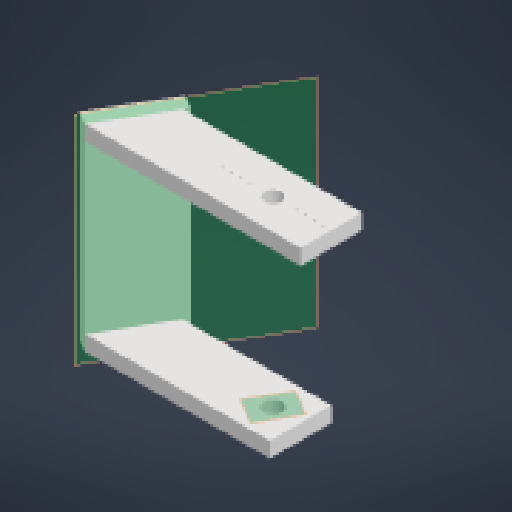
# Autodesk Inventor part: manipulator_arm
Saved by Autodesk Inventor 2024 (Build 280153000, 153)
## iProperties
Created: 2023-05-17
Part Number: manipulator_arm
Material: Типовые
Document SubType Name: Modeling
Designer: user
Density: 1 g/cm^3
Appearance: По умолчанию
Author: user
Autodesk Inventor part; units mm, degrees
ref_plane "YZ Plane" through (0, 0, 0) normal (1, 0, 0) x (0, 1, 0)
ref_plane "XZ Plane" through (0, 0, 0) normal (0, 1, 0) x (-1, 0, 0)
ref_plane "XY Plane" through (0, 0, 0) normal (0, 0, 1) x (1, 0, 0)
sketch "Эскиз1" plane through (0, 0, 0) normal (0, 0, 1) x (1, 0, 0)
  line L0 (-81, 10) -> (19, 10)
  line L1 (19, 10) -> (19, -10)
  line L2 (19, -10) -> (-81, -10)
  line L3 (-81, -10) -> (-81, 10)
  line L4 (19, 0) -> (0, 0) construction
  arc A0 (16.8881, -2.4697) -> (16.8881, 2.4697) centre (16.5, 0) ccw construction
  circle A1 centre (16.5, 0) radius 0.65 construction
  circle A2 centre (13.5, 0) radius 0.65 construction
  circle A3 centre (10.5, 0) radius 0.65 construction
  circle A4 centre (7.5, 0) radius 0.65 construction
  circle A5 centre (-7.5, 0) radius 0.65 construction
  circle A6 centre (-10.5, 0) radius 0.65 construction
  circle A7 centre (-13.5, 0) radius 0.65 construction
  circle A8 centre (-16.5, 0) radius 0.65 construction
  circle A9 centre (-16.5, 0) radius 0.4
  circle A10 centre (-13.5, 0) radius 0.4
  circle A11 centre (-10.5, 0) radius 0.4
  circle A12 centre (-7.5, 0) radius 0.4
  circle A13 centre (7.5, 0) radius 0.4
  circle A14 centre (10.5, 0) radius 0.4
  circle A15 centre (13.5, 0) radius 0.4
  circle A16 centre (16.5, 0) radius 0.4
  circle A17 centre (0, 0) radius 2.75 projected
  dimension "d0" = 20
  dimension "d3" = 100
  dimension "d28" = 0.8
  constraints: 10 end point, 8 centre point, 8 coincident, 7 equal radius, 3 perpendicular, 1 horizontal, 1 midpoint, 1 parallel, 1 tangent
  measures "d0" distance of L0.end L1.end
  measures "d3" distance of L1.end L2.end
  measures "d28" diameter of A9
extrude "Выдавливание1" add sketch "Эскиз1" along normal blind 5
ref_plane "РабПлоскость1" through (0, 0, -54.2) normal (0, 0, -1) x (-0.5, -0.8660254, 0)
sketch "Эскиз2" plane through (0, 0, -54.2) normal (0, 0, -1) x (-0.5, -0.8660254, 0)
  line L0 (31.8397, 75.1481) -> (49.1603, 65.1481) projected
  line L1 (49.1603, 65.1481) -> (4.1603, -12.7942)
  line L2 (49.1603, 65.1481) -> (-0.8397, -21.4545) projected
  line L3 (4.1603, -12.7942) -> (-13.1603, -2.7942)
  line L4 (-18.1603, -11.4545) -> (31.8397, 75.1481) projected
  line L5 (-13.1603, -2.7942) -> (31.8397, 75.1481)
  circle A0 centre (0, 0) radius 3 projected
  point P0 (0, 0)
  dimension "d4" = 90
  constraints: 6 end point, 2 point on line, 1 collinear, 1 perpendicular
  measures "d4" distance of L0.end L1.end
extrude "Выдавливание2" add sketch "Эскиз2" along normal blind 5
ref_plane "РабПлоскость3" through (-81, -10, 5) normal (-0.8660254, 0.5, 0) x (0.5, 0.8660254, 0)
ref_plane "РабПлоскость2" through (-22.6159, -10.6718, -31.45) normal (-0.8660254, 0.5, 0) x (0.5, 0.8660254, 0)
sketch "Эскиз3" plane through (-81, -10, 5) normal (-0.8660254, 0.5, 0) x (0.5, 0.8660254, 0)
  line L0 (0, 59.2) -> (17.3205, 59.2) projected
  line L1 (0, 5) -> (50, 5) projected
  line L2 (0, 59.2) -> (25, 59.2)
  line L3 (25, 59.2) -> (25, 5)
  line L4 (25, 5) -> (0, 5)
  line L5 (0, 5) -> (0, 59.2)
  point P0 (49.1603, 5)
  point P1 (0, 5)
  point P2 (17.3205, 59.2)
  dimension "d7" = 25
  constraints: 8 end point, 2 parallel, 1 horizontal, 1 midpoint, 1 perpendicular
  measures "d7" distance of L1.start L3.end
extrude "Выдавливание3" add sketch "Эскиз3" along normal blind 5
move faces "Перенос1" translate (0, 0, 5) faces at (-82.4434, -5.8333, 0)
move faces "Перенос2" translate (0, 0, -5) faces at (-82.4434, -5.8333, -54.2)
move faces "Перенос3" translate (0, 0, -6.5) faces at (-79.0755, 6.6667, -54.2)
move faces "Перенос4" translate (0, 0, 7.5) faces at (-79.0755, 6.6667, 0)
move faces "Перенос5" translate (0, 0, 5) faces at (-72.5032, 11.3835, 0)
move faces "Перенос6" translate (0, 0, -5) faces at (-72.5032, 11.3835, -54.2)
sketch "Эскиз4" plane through (-85.3301, -7.5, 5) normal (-0.8660254, 0.5, 0) x (0, 0, 1)
  line L0 (0, 25) -> (-64.2, 25) projected
  line L1 (-57.1, 25) -> (-7.1, 25)
  line L2 (-7.1, 25) -> (-7.1, 8)
  line L3 (-7.1, 8) -> (-57.1, 8)
  line L4 (-57.1, 8) -> (-57.1, 25)
  line L5 (-64.2, 0) -> (0, 0) projected
  point P0 (-5, 49.1603)
  point P1 (-32.1, 8)
  point P2 (-32.1, 0)
  point P3 (-7.1, 25)
  dimension "d29" = 17
  dimension "d30" = 50
  constraints: 8 end point, 2 midpoint, 2 parallel, 1 horizontal, 1 perpendicular, 1 point on line, 1 vertical alignment
  measures "d29" distance of L1.end L2.end
  measures "d30" distance of L2.end L3.end
extrude "Выдавливание4" cut sketch "Эскиз4" against normal blind 5
